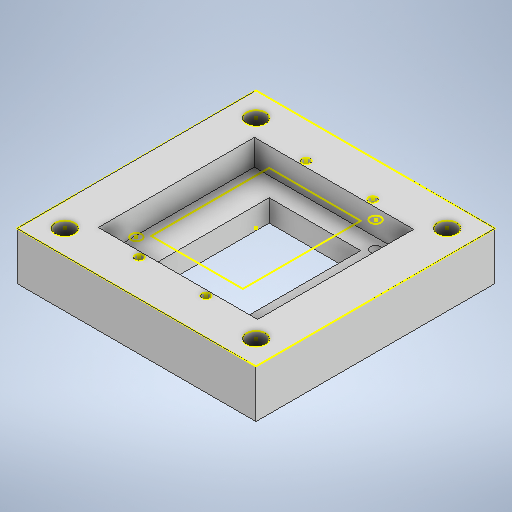
# Autodesk Inventor part: dmd_cnc
Saved by Autodesk Inventor 2025.1 (Build 291241000, 241)
## iProperties
Created: 2024-10-23
Part Number: dmd_cnc
Material: Ogólny
Document SubType Name: Modeling
Designer: PC
Density: 1 g/cm^3
Appearance: Domyślna
Author: PC
Autodesk Inventor part; units mm, degrees
ref_plane "YZ Plane" through (0, 0, 0) normal (1, 0, 0) x (0, 1, 0)
ref_plane "XZ Plane" through (0, 0, 0) normal (0, 1, 0) x (-1, 0, 0)
ref_plane "XY Plane" through (0, 0, 0) normal (0, 0, 1) x (1, 0, 0)
sketch "Baza" plane through (0, 0, 0) normal (0, 1, 0) x (-1, 0, 0)
  line L0 (30, 30) -> (-30, 30) construction
  line L1 (-30, 30) -> (-30, -30) construction
  line L2 (-30, -30) -> (30, -30) construction
  line L3 (30, -30) -> (30, 30) construction
  line L4 (30, 30) -> (-30, -30) construction
  line L5 (-30, 30) -> (30, -30) construction
  circle A0 centre (30, -30) radius 3
  circle A1 centre (30, 30) radius 3
  circle A2 centre (-30, 30) radius 3
  circle A3 centre (-30, -30) radius 3
  line L6 (37.5, 37.5) -> (-37.5, 37.5)
  line L7 (-37.5, 37.5) -> (-37.5, -37.5)
  line L8 (-37.5, -37.5) -> (37.5, -37.5)
  line L9 (37.5, -37.5) -> (37.5, 37.5)
  line L10 (37.5, 37.5) -> (-37.5, -37.5) construction
  line L11 (-37.5, 37.5) -> (37.5, -37.5) construction
  line L12 (10.475, 26.2) -> (-10.475, 26.2) construction
  line L13 (-10.475, 26.2) -> (-10.475, -26.2) construction
  line L14 (-10.475, -26.2) -> (10.475, -26.2) construction
  line L15 (10.475, -26.2) -> (10.475, 26.2) construction
  line L16 (10.475, 26.2) -> (-10.475, -26.2) construction
  line L17 (-10.475, 26.2) -> (10.475, -26.2) construction
  circle A4 centre (10.475, 26.2) radius 1.25
  circle A5 centre (-10.475, 26.2) radius 1.25
  circle A6 centre (-10.475, -26.2) radius 1.25
  circle A7 centre (10.475, -26.2) radius 1.25
  line L18 (14.375, 18.5) -> (-14.375, 18.5)
  line L19 (-14.375, 18.5) -> (-14.375, -18.5)
  line L20 (-14.375, -18.5) -> (14.375, -18.5)
  line L21 (14.375, -18.5) -> (14.375, 18.5)
  line L22 (14.375, 18.5) -> (-14.375, -18.5) construction
  line L23 (-14.375, 18.5) -> (14.375, -18.5) construction
  circle A8 centre (16.413, 21.1229) radius 1.6
  circle A9 centre (-16.413, -21.1229) radius 1.6
  line L24 (16.413, 21.1229) -> (-16.413, -21.1229) construction
  point P0 (0, 0)
  dimension "d0" = 60
  dimension "d1" = 6
  dimension "d2" = 75
  dimension "d3" = 20.95
  dimension "d4" = 52.4
  dimension "d5" = 2.5
  dimension "d6" = 28.75
  dimension "d7" = 37
  dimension "d12" = 3.2
  dimension "d13" = 53.5
  dimension "d14" = 26.75
  constraints: 50 end point, 10 centre point, 9 midpoint, 8 coincident, 8 parallel, 7 equal radius, 6 perpendicular, 4 horizontal, 1 collinear
  measures "d0" distance of L1.end L2.end
  measures "d1" diameter of A0
  measures "d2" distance of L8.end L7.end
  measures "d3" distance of L13.end L14.end
  measures "d4" distance of L14.end L12.start
  measures "d5" diameter of A4
  measures "d6" distance of L20.end L19.end
  measures "d7" distance of L18.end L19.end
  measures "d12" diameter of A8
  measures "d13" distance of L24.end L24.start
  measures "d14" distance of point (0, 0) L24.start
extrude "Wyciągnięcie proste1" add sketch "Baza" along normal blind 15
sketch "Szkic2" plane through (0, 15, 0) normal (0, 1, 0) x (1, 0, 0)
  line L0 (37.5, -37.5) -> (37.5, 37.5) projected
  line L1 (37.5, 37.5) -> (-37.5, 37.5) projected
  line L2 (-37.5, 37.5) -> (-37.5, -37.5) projected
  line L3 (-37.5, -37.5) -> (37.5, -37.5) projected
  circle A0 centre (16.413, 21.1229) radius 1.6 projected
  circle A1 centre (-10.475, 26.2) radius 1.25 projected
  circle A2 centre (10.475, 26.2) radius 1.25 projected
  circle A3 centre (10.475, -26.2) radius 1.25 projected
  circle A4 centre (-10.475, -26.2) radius 1.25 projected
  circle A5 centre (30, 30) radius 3 projected
  circle A6 centre (30, -30) radius 3 projected
  circle A7 centre (-30, -30) radius 3 projected
  circle A8 centre (-30, 30) radius 3 projected
  circle A9 centre (-16.413, -21.1229) radius 1.6 projected
  line L4 (-14.375, -18.5) -> (-14.375, 18.5) projected
  line L5 (-14.375, 18.5) -> (14.375, 18.5) projected
  line L6 (14.375, 18.5) -> (14.375, -18.5) projected
  line L7 (14.375, -18.5) -> (-14.375, -18.5) projected
  line L8 (-14.375, -18.5) -> (-14.375, 18.5) projected
  point P0 (0, 0)
sketch "Szkic3" plane through (0, 15, 0) normal (0, 1, 0) x (1, 0, 0)
  line L0 (25, -24.5) -> (-25, -24.5)
  line L1 (-25, -24.5) -> (-25, 24.5)
  line L2 (-25, 24.5) -> (25, 24.5)
  line L3 (25, 24.5) -> (25, -24.5)
  line L4 (25, -24.5) -> (-25, 24.5) construction
  line L5 (-25, -24.5) -> (25, 24.5) construction
  point P0 (0, 0)
  dimension "d16" = 49
  dimension "d17" = 50
  constraints: 12 end point, 2 midpoint, 2 parallel, 1 horizontal, 1 perpendicular
  measures "d16" distance of L0.end L1.end
  measures "d17" distance of L1.end L2.end
extrude "Wyciągnięcie proste2" cut sketch "Szkic3" against normal blind 8.1
